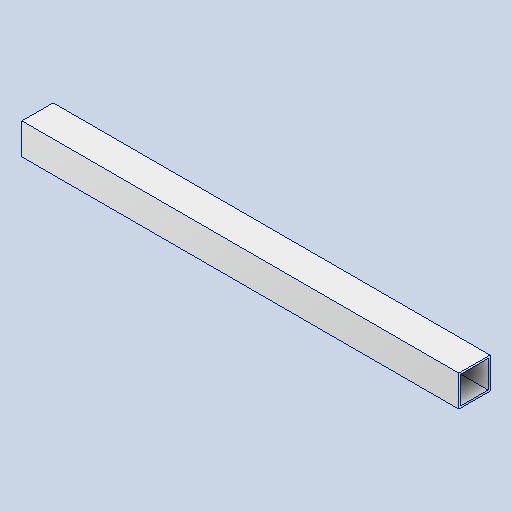
# Autodesk Inventor part: Part1-17-13.31255in
Saved by Autodesk Inventor 2025.1 (Build 291241020, 241B)
## iProperties
Created: 2023-03-16
Part Number: Part1-17-13.31255in
Material: Aluminum 6061
Document SubType Name: Modeling
Designer: mvp5338
Density: 2.7 g/cm^3
Appearance: Aluminum - Flat
Author: mvp5338
Autodesk Inventor part; units mm, degrees
ref_plane "YZ Plane" through (0, 0, 0) normal (1, 0, 0) x (0, 1, 0)
ref_plane "XZ Plane" through (0, 0, 0) normal (0, 1, 0) x (-1, 0, 0)
ref_plane "XY Plane" through (0, 0, 0) normal (0, 0, 1) x (1, 0, 0)
sketch "Sketch1" plane through (0, 0, 0) normal (1, 0, 0) x (0, 1, 0)
  line L0 (12.7, 12.2788) -> (-12.7, 12.2788)
  line L1 (-12.7, 12.2788) -> (-12.7, -13.1212)
  line L2 (-12.7, -13.1212) -> (12.7, -13.1212)
  line L3 (12.7, -13.1212) -> (12.7, 12.2788)
  line L4 (0, 32.4321) -> (0, -31.5519)
  line L5 (24.3369, 0) -> (-19.9975, 0)
  line L6 (11.1125, -11.5337) -> (-11.1125, -11.5337)
  line L7 (-11.1125, -11.5337) -> (-11.1125, 10.6913)
  line L8 (-11.1125, 10.6913) -> (11.1125, 10.6913)
  line L9 (11.1125, 10.6913) -> (11.1125, -11.5337)
  point P0 (0, 0)
  dimension "d0" = 25.4
  dimension "d24" = 1.5875
  dimension "d25" = 1.5875
  dimension "d26" = 1.5875
  dimension "d27" = 1.5875
  constraints: 20 end point, 4 parallel, 3 horizontal, 3 perpendicular, 1 vertical, 1 other
  measures "d0" distance of L2.end L0.start
  measures "d24" distance between parallel lines of L2 L6
  measures "d25" distance between parallel lines of L0 L8
  measures "d26" distance between parallel lines of L1 L7
  measures "d27" distance between parallel lines of L3 L9
extrude "Extrusion1" add sketch "Sketch1" along normal blind 355.6 contours L3 L5 L9 L8 L4 L0 | L4 L8 L7 L5 L1 L0 | L3 L2 L4 L6 L9 L5 | L5 L7 L6 L4 L2 L1
equation "\"d25\" = d24"
equation "\"d26\" = d24"
equation "\"d27\" = d26"
body "Solid1"
